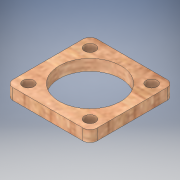
# Autodesk Inventor part: BearingMount
Saved by Autodesk Inventor 2019 (Build 230136000, 136)
## iProperties
Created: 2019-01-18
Part Number: BearingMount
Material: Wood (Birch)
Document SubType Name: Modeling
Designer: nxgam
Density: 0.55 g/cm^3
Appearance: Birch - Natural Polished
Author: nxgam
Autodesk Inventor part; units mm, degrees
ref_plane "YZ Plane" through (0, 0, 0) normal (1, 0, 0) x (0, 1, 0)
ref_plane "XZ Plane" through (0, 0, 0) normal (0, 1, 0) x (-1, 0, 0)
ref_plane "XY Plane" through (0, 0, 0) normal (0, 0, 1) x (1, 0, 0)
sketch "Sketch1" plane through (0, 0, 0) normal (0, 1, 0) x (-1, 0, 0)
  circle A0 centre (0, 0) radius 13.97
  line L0 (-19.05, 19.05) -> (19.05, 19.05)
  line L1 (19.05, 19.05) -> (19.05, -19.05)
  line L2 (19.05, -19.05) -> (-19.05, -19.05)
  line L3 (-19.05, -19.05) -> (-19.05, 19.05)
  line L4 (-19.05, 19.05) -> (19.05, -19.05) construction
  line L5 (19.05, 19.05) -> (-19.05, -19.05) construction
  dimension "d0" = 27.94
  dimension "d1" = 38.1
  dimension "d2" = 38.1
  constraints: 12 end point, 2 midpoint, 2 parallel, 1 centre point, 1 coincident, 1 horizontal, 1 perpendicular
  measures "d0" diameter of A0
  measures "d1" distance of L1.end L2.end
  measures "d2" distance of L0.end L1.end
extrude "Extrusion1" add sketch "Sketch1" along normal blind 5.08
sketch "Sketch2" plane through (0, 5.08, 0) normal (0, 1, 0) x (1, 0, 0)
  circle A0 centre (0, 0) radius 13.97 construction
  line L0 (-19.05, -19.05) -> (-19.05, 19.05) construction
  line L1 (-19.05, 19.05) -> (19.05, 19.05) construction
  line L2 (19.05, 19.05) -> (19.05, -19.05) construction
  line L3 (19.05, -19.05) -> (-19.05, -19.05) construction
  line L4 (-19.05, -19.05) -> (0, 0) construction
  point P0 (-13.97, -13.97)
  point P1 (13.97, -13.97)
  point P2 (13.97, 13.97)
  point P3 (-13.97, 13.97)
  dimension "d5" = 13.97
  dimension "d8" = 360
  constraints: 2 end point, 1 point on line, 5 other
  measures "d5" horizontal distance of point (0, 0) point (-13.97, -13.97)
hole "Hole1" at (-13.97, 5.08, 13.97) at (13.97, 5.08, 13.97) at (13.97, 5.08, -13.97) at (-13.97, 5.08, -13.97) direction (0, -1, 0) diameter 5 end through all
fillet "Fillet1" radius 3.175 4 edges at (-19.05, 2.54, 19.05) (-19.05, 2.54, -19.05) (19.05, 2.54, -19.05) (19.05, 2.54, 19.05)
equation "\"d2\" = d1"
body "Solid1"
